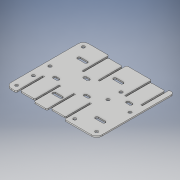
# Autodesk Inventor part: Tier2Plate
Saved by Autodesk Inventor 2018 (Build 220112000, 112)
## iProperties
Created: 2019-03-26
Part Number: Tier2Plate
Material: Generic
Document SubType Name: Modeling
Designer: anirudh
Density: 1 g/cm^3
Appearance: Default
Author: anirudh
Autodesk Inventor part; units mm, degrees
ref_plane "YZ Plane" through (0, 0, 0) normal (1, 0, 0) x (0, 1, 0)
ref_plane "XZ Plane" through (0, 0, 0) normal (0, 1, 0) x (-1, 0, 0)
ref_plane "XY Plane" through (0, 0, 0) normal (0, 0, 1) x (1, 0, 0)
sketch "Sketch4" plane through (0, 0, 0) normal (0, 1, 0) x (-1, 0, 0)
  line L0 (0, 0) -> (116.84, 0)
  line L1 (116.84, 0) -> (116.84, -91.44)
  line L2 (116.84, -91.44) -> (0, -91.44)
  line L3 (0, -91.44) -> (0, 0)
  dimension "d17" = 116.84
  dimension "d18" = 91.44
  constraints: 8 end point, 2 parallel, 1 horizontal, 1 perpendicular
  measures "d17" distance of L1.end L2.end
  measures "d18" distance of L0.end L1.end
extrude "Extrusion4" add sketch "Sketch4" along normal blind 1.5875
fillet "Fillet3" radius 6.35 4 edges at (0, 0.7937, 0) (0, 0.7937, -91.44) (-116.84, 0.7937, 0) (-116.84, 0.7937, -91.44)
sketch "Sketch5" plane through (0, 1.5875, 0) normal (0, 1, 0) x (1, 0, 0)
  arc A0 (-116.84, 6.35) -> (-110.49, 0) centre (-110.49, 6.35) ccw projected
  circle A1 centre (-110.49, 6.35) radius 1.8
  arc A2 (-110.49, 91.44) -> (-116.84, 85.09) centre (-110.49, 85.09) ccw projected
  circle A3 centre (-110.49, 85.09) radius 1.8
  circle A4 centre (-41.91, 6.35) radius 1.8
  circle A5 centre (-41.91, 61.0616) radius 1.8
  point P0 (0, 0)
  dimension "d22" = 3.6
  dimension "d23" = 3.6
  dimension "d27" = 3.6
  dimension "d28" = 3.6
  constraints: 4 centre point, 2 coincident
  measures "d22" diameter of A1
  measures "d23" diameter of A3
  measures "d27" diameter of A4
  measures "d28" diameter of A5
extrude "Extrusion5" cut sketch "Sketch5" against normal blind 1.5875
sketch "Sketch6" plane through (0, 1.5875, 0) normal (0, 1, 0) x (1, 0, 0)
  arc A0 (-116.84, 6.35) -> (-110.49, 0) centre (-110.49, 6.35) ccw projected
  line L0 (-102.9208, 3.048) -> (-102.9208, 31.75)
  line L1 (-102.9208, 31.75) -> (-104.8258, 31.75)
  line L2 (-104.8258, 31.75) -> (-104.8258, 0)
  line L3 (-102.9208, 3.048) -> (-102.9208, 31.75)
  line L4 (-85.8266, 31.75) -> (-83.9216, 31.75)
  line L5 (-83.9216, 31.75) -> (-83.9216, 0)
  line L6 (-85.8266, 3.048) -> (-85.8266, 31.75)
  line L7 (-110.49, 0) -> (-6.35, 0) projected
  line L8 (-85.8266, 3.048) -> (-102.9208, 3.048)
  circle A1 centre (-41.91, 6.35) radius 1.8 projected
  line L9 (-41.91, 6.35) -> (-47.5742, 6.35)
  line L10 (-47.5742, 6.35) -> (-47.5742, 0)
  line L11 (-47.5742, 6.35) -> (-47.5742, 31.75)
  line L12 (-47.5742, 31.75) -> (-49.4792, 31.75)
  line L13 (-47.5742, 0) -> (-47.5742, 31.75)
  line L14 (-66.5734, 31.75) -> (-68.4784, 31.75)
  line L15 (-68.4784, 31.75) -> (-68.4784, 0)
  line L16 (-66.5734, 3.048) -> (-66.5734, 31.75)
  line L17 (-49.4792, 3.048) -> (-66.5734, 3.048)
  line L18 (-102.9208, 0) -> (-85.8266, 0)
  line L19 (-66.5734, 0) -> (-49.4792, 0)
  line L20 (-104.8258, 0) -> (-83.9216, 0)
  line L21 (-68.4784, 0) -> (-47.5742, 0)
  line L22 (-49.4792, 3.048) -> (-49.4792, 31.75)
  line L23 (-83.9216, 0) -> (-83.9216, 20.3962)
  arc A2 (-80.3944, 22.1962) -> (-80.3944, 18.5962) centre (-80.3944, 20.3962) ccw
  arc A3 (-72.0056, 18.5962) -> (-72.0056, 22.1962) centre (-72.0056, 20.3962) ccw
  line L24 (-80.3944, 18.5962) -> (-72.0056, 18.5962)
  line L25 (-72.0056, 22.1962) -> (-80.3944, 22.1962)
  point P0 (0, 0)
  dimension "d33" = 31.75
  dimension "d35" = 17.0942
  dimension "d37" = 3.048
  dimension "d38" = 5.6642
  dimension "d40" = 17.0942
  dimension "d42" = 3.048
  constraints: 50 end point, 9 horizontal, 6 perpendicular, 5 parallel, 4 point on circle, 4 point on line, 2 centre point, 2 tangent, 2 vertical, 8 other
  measures "d33" distance of L18.start L0.end
  measures "d35" distance of L0.end L4.start
  measures "d37" distance of L6.start L18.end
  measures "d38" distance of L9.start L9.end
  measures "d40" distance of L12.end L14.start
  measures "d42" distance of L19.end L17.start
extrude "Extrusion6" cut sketch "Sketch6" against normal blind 1.5875 contours L8 L6 L4 L5 L7 L2 L1 L0 | L15 L14 L16 L17 L22 L12 L11 L10 L7 | L25 A3 L24 A2
fillet "Fillet4" radius 1.5875 7 edges at (-102.9208, 0.7937, -3.048) (-85.8266, 0.7937, -3.048) (-83.9216, 0.7937, 0) (-68.4784, 0.7937, 0) (-66.5734, 0.7937, -3.048) (-49.4792, 0.7937, -3.048) (-47.5742, 0.7937, 0)
fillet "Fillet5" radius 1.5875 1 edges at (-104.8258, 0.7937, 0)
sketch "Sketch7" plane through (0, 1.5875, 0) normal (0, 1, 0) x (1, 0, 0)
  line L0 (-116.84, 85.09) -> (-116.84, 6.35) projected
  line L1 (-110.49, 91.44) -> (-6.35, 91.44) projected
  line L2 (-84.7471, 88.392) -> (-84.7471, 59.69)
  line L3 (-84.7471, 59.69) -> (-86.6521, 59.69)
  line L4 (-86.6521, 59.69) -> (-86.6521, 91.44)
  line L5 (-67.6529, 59.69) -> (-65.7479, 59.69)
  line L6 (-65.7479, 59.69) -> (-65.7479, 91.44)
  line L7 (-84.7471, 88.392) -> (-67.6529, 88.392)
  line L8 (-86.6521, 91.44) -> (-65.7479, 91.44)
  line L9 (-67.6529, 88.392) -> (-67.6529, 59.69)
  line L10 (-84.7471, 88.392) -> (-84.7471, 59.69)
  point P0 (0, 0)
  dimension "d55" = 17.0942
  constraints: 18 end point, 3 perpendicular, 2 horizontal, 2 parallel, 2 point on line
  measures "d55" distance of L2.end L5.start
extrude "Extrusion7" cut sketch "Sketch7" against normal blind 1.5875
sketch "Sketch8" plane through (0, 1.5875, 0) normal (0, 1, 0) x (1, 0, 0)
  line L0 (-86.6521, 59.69) -> (-86.6521, 91.44) projected
  line L1 (-86.6521, 91.44) -> (-110.49, 91.44) projected
  arc A0 (-93.1291, 69.2438) -> (-93.1291, 72.8438) centre (-93.1291, 71.0438) ccw
  arc A1 (-101.5111, 72.8438) -> (-101.5111, 69.2438) centre (-101.5111, 71.0438) ccw
  line L2 (-101.5111, 69.2438) -> (-93.1291, 69.2438)
  line L3 (-93.1291, 72.8438) -> (-101.5111, 72.8438)
  line L4 (-67.6529, 88.392) -> (-84.7471, 88.392) projected
  arc A2 (-59.2709, 72.8438) -> (-59.2709, 69.2438) centre (-59.2709, 71.0438) ccw
  arc A3 (-50.8889, 69.2438) -> (-50.8889, 72.8438) centre (-50.8889, 71.0438) ccw
  line L5 (-50.8889, 69.2438) -> (-59.2709, 69.2438)
  line L6 (-59.2709, 72.8438) -> (-50.8889, 72.8438)
  point P0 (0, 0)
  dimension "d63" = 3.6
  dimension "d64" = 3.6
  constraints: 8 end point, 8 point on circle, 4 centre point, 1 horizontal, 1 parallel
  measures "d63" diameter of A0
  measures "d64" diameter of A1
extrude "Extrusion8" cut sketch "Sketch8" against normal blind 1.5875
fillet "Fillet6" radius 1.5875 4 edges at (-65.7479, 0.7937, -91.44) (-67.6529, 0.7937, -88.392) (-84.7471, 0.7937, -88.392) (-86.6521, 0.7937, -91.44)
sketch "Sketch9" plane through (0, 1.5875, 0) normal (0, 1, 0) x (1, 0, 0)
  circle A0 centre (-41.91, 61.0616) radius 1.8 projected
  line L0 (-36.2458, 91.44) -> (-36.2458, 59.69)
  line L1 (-36.2458, 59.69) -> (-34.3408, 59.69)
  line L2 (-34.3408, 59.69) -> (-34.3408, 88.392)
  line L3 (-36.2458, 91.44) -> (-36.2458, 59.69)
  line L4 (-17.2466, 59.69) -> (-15.3416, 59.69)
  line L5 (-15.3416, 59.69) -> (-15.3416, 91.44)
  line L6 (-17.2466, 88.392) -> (-17.2466, 59.69)
  line L7 (-64.1604, 91.44) -> (-6.35, 91.44) projected
  line L8 (-17.2466, 88.392) -> (-34.3408, 88.392)
  line L9 (-36.2458, 91.44) -> (-15.3416, 91.44)
  line L10 (-6.35, 0) -> (-45.9867, 0) projected
  arc A1 (-29.9847, 22.1962) -> (-29.9847, 18.5962) centre (-29.9847, 20.3962) ccw
  arc A2 (-21.6027, 18.5962) -> (-21.6027, 22.1962) centre (-21.6027, 20.3962) ccw
  line L11 (-21.6027, 18.5962) -> (-29.9847, 18.5962)
  line L12 (-29.9847, 22.1962) -> (-21.6027, 22.1962)
  point P0 (0, 0)
  dimension "d70" = 31.75
  dimension "d72" = 17.0942
  dimension "d78" = 3.6
  dimension "d79" = 3.6
  constraints: 22 end point, 4 point on circle, 3 horizontal, 3 parallel, 3 perpendicular, 2 centre point, 2 point on line, 1 tangent, 1 vertical
  measures "d70" distance of L0.start L0.end
  measures "d72" distance of L1.end L4.start
  measures "d78" diameter of A1
  measures "d79" diameter of A2
extrude "Extrusion9" cut sketch "Sketch9" against normal blind 1.5875 contours L7 L5 L4 L6 L8 L2 L1 L0 | L12 A2 L11 A1
fillet "Fillet7" radius 1.5875 4 edges at (-17.2466, 0.7937, -88.392) (-15.3416, 0.7937, -91.44) (-34.3408, 0.7937, -88.392) (-36.2458, 0.7937, -91.44)
sketch "Sketch10" plane through (0, 1.5875, 0) normal (0, 1, 0) x (1, 0, 0)
  line L0 (-15.3416, 59.69) -> (-15.3416, 89.8525) projected
  line L1 (-9.6774, 59.69) -> (-9.6774, -28.742)
  line L2 (-9.6774, -28.742) -> (4.8684, -28.742)
  line L3 (4.8684, -28.742) -> (4.8684, 98.8389)
  line L4 (4.8684, 98.8389) -> (-9.6774, 98.8389)
  line L5 (-9.6774, 98.8389) -> (-9.6774, -28.742)
  point P0 (0, 0)
  dimension "d83" = 5.6642
  constraints: 10 end point, 2 parallel, 1 horizontal, 1 perpendicular
  measures "d83" distance of L0.start L1.start
extrude "Extrusion10" cut sketch "Sketch10" against normal blind 1.5875
fillet "Fillet8" radius 6.35 1 edges at (-9.6774, 0.7937, 0)
fillet "Fillet9" radius 3.175 1 edges at (-9.6774, 0.7937, -91.44)
sketch "Sketch11" plane through (0, 1.5875, 0) normal (0, 1, 0) x (1, 0, 0)
  line L0 (-102.9208, 31.75) -> (-104.8258, 31.75) projected
  line L1 (-85.8266, 31.75) -> (-85.8266, 4.6355) projected
  arc A0 (-96.1737, 38.63) -> (-96.1737, 35.03) centre (-96.1737, 36.83) ccw
  arc A1 (-92.5737, 35.03) -> (-92.5737, 38.63) centre (-92.5737, 36.83) ccw
  line L2 (-96.1737, 35.03) -> (-92.5737, 35.03)
  line L3 (-92.5737, 38.63) -> (-96.1737, 38.63)
  line L4 (-84.7471, 86.8045) -> (-84.7471, 59.69) projected
  line L5 (-67.6529, 86.8045) -> (-67.6529, 59.69) projected
  arc A2 (-78, 56.41) -> (-78, 52.81) centre (-78, 54.61) ccw
  arc A3 (-74.4, 52.81) -> (-74.4, 56.41) centre (-74.4, 54.61) ccw
  line L6 (-78, 52.81) -> (-74.4, 52.81)
  line L7 (-74.4, 56.41) -> (-78, 56.41)
  line L8 (-66.5734, 4.6355) -> (-66.5734, 31.75) projected
  line L9 (-49.4792, 31.75) -> (-49.4792, 4.6355) projected
  arc A4 (-59.8263, 38.63) -> (-59.8263, 35.03) centre (-59.8263, 36.83) ccw
  arc A5 (-56.2263, 35.03) -> (-56.2263, 38.63) centre (-56.2263, 36.83) ccw
  line L10 (-59.8263, 35.03) -> (-56.2263, 35.03)
  line L11 (-56.2263, 38.63) -> (-59.8263, 38.63)
  line L12 (-34.3408, 59.69) -> (-34.3408, 86.8045) projected
  line L13 (-17.2466, 86.8045) -> (-17.2466, 59.69) projected
  arc A6 (-27.5937, 56.41) -> (-27.5937, 52.81) centre (-27.5937, 54.61) ccw
  arc A7 (-23.9937, 52.81) -> (-23.9937, 56.41) centre (-23.9937, 54.61) ccw
  line L14 (-27.5937, 52.81) -> (-23.9937, 52.81)
  line L15 (-27.5937, 56.41) -> (-23.9937, 56.41)
  point P0 (0, 0)
  dimension "d90" = 3.6
  dimension "d91" = 3.6
  dimension "d94" = 3.6
  dimension "d95" = 3.6
  dimension "d99" = 3.6
  dimension "d100" = 3.6
  dimension "d103" = 3.6
  dimension "d104" = 3.6
  constraints: 16 end point, 16 point on circle, 8 centre point, 6 tangent, 4 horizontal, 4 parallel
  measures "d90" diameter of A0
  measures "d91" diameter of A1
  measures "d94" diameter of A2
  measures "d95" diameter of A3
  measures "d99" diameter of A4
  measures "d100" diameter of A5
  measures "d103" diameter of A6
  measures "d104" diameter of A7
extrude "Extrusion11" cut sketch "Sketch11" against normal blind 1.5875
sketch "Sketch12" plane through (0, 1.5875, 0) normal (0, 1, 0) x (1, 0, 0)
  circle A0 centre (-110.49, 6.35) radius 1.8 projected
  circle A1 centre (-110.49, 85.09) radius 1.8 projected
  circle A2 centre (-41.91, 6.35) radius 1.8 projected
  circle A3 centre (-41.91, 61.0616) radius 1.8 projected
  circle A4 centre (-110.49, 45.72) radius 1.8
  circle A5 centre (-41.91, 45.72) radius 1.8
  point P0 (0, 0)
  dimension "d107" = 3.6
  dimension "d108" = 3.6
  constraints: 2 centre point
  measures "d107" diameter of A4
  measures "d108" diameter of A5
extrude "Extrusion12" cut sketch "Sketch12" against normal blind 1.5875 contours A4 | A5
sketch "Sketch13" plane through (0, 1.5875, 0) normal (0, 1, 0) x (1, 0, 0)
  circle A0 centre (-110.49, 6.35) radius 1.8 projected
  circle A1 centre (-110.49, 45.72) radius 1.8 projected
  circle A2 centre (-110.49, 85.09) radius 1.8 projected
  circle A3 centre (-41.91, 6.35) radius 1.8 projected
  arc A4 (-16.0274, 0) -> (-9.6774, 6.35) centre (-16.0274, 6.35) ccw projected
  circle A5 centre (-41.91, 45.72) radius 1.8 projected
  circle A6 centre (-16.0274, 6.35) radius 1.8
  circle A7 centre (-16.0274, 45.72) radius 1.8
  circle A8 centre (-41.91, 61.0616) radius 1.8 projected
  line L0 (-64.1604, 91.44) -> (-37.8333, 91.44) projected
  circle A9 centre (-110.49, 26.035) radius 1.8
  point P0 (0, 0)
  dimension "d111" = 3.6
  dimension "d112" = 3.6
  dimension "d115" = 3.6
  constraints: 3 centre point, 1 coincident
  measures "d111" diameter of A6
  measures "d112" diameter of A7
  measures "d115" diameter of A9
extrude "Extrusion14" cut sketch "Sketch13" against normal blind 1.5875 contours A6 | A7 | A9
body "Solid2"
